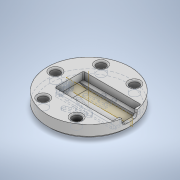
# Autodesk Inventor part: hmmb
Saved by Autodesk Inventor 2021 (Build 250183000, 183)
## iProperties
Created: 2020-07-09
Part Number: hmmb
Material: Generic
Document SubType Name: Modeling
Designer: andre
Density: 1 g/cm^3
Appearance: Default
Author: andre
## iProperties of the stored document _3DPrint.ipt
Created: 2020-07-09
Part Number: _3DPrint
Material: Generic
Document SubType Name: Modeling
Designer: andre
Density: 1 g/cm^3
Appearance: Default
Author: andre
Autodesk Inventor part; units mm, degrees
ref_plane "YZ Plane" through (0, 0, 0) normal (1, 0, 0) x (0, 1, 0)
ref_plane "XZ Plane" through (0, 0, 0) normal (0, 1, 0) x (-1, 0, 0)
ref_plane "XY Plane" through (0, 0, 0) normal (0, 0, 1) x (1, 0, 0)
sketch "Sketch1" plane through (0, 0, 0) normal (0, 1, 0) x (-1, 0, 0)
  circle A0 centre (0, 0) radius 26
  dimension "d0" = 52
  constraints: 1 centre point
  measures "d0" diameter of A0
extrude "Extrusion1" add sketch "Sketch1" along normal blind 8
chamfer "Chamfer2" distance 1.6 angle 45 1 edges at (26, 0, 0)
sketch "Sketch2" plane through (0, 8, 0) normal (0, 1, 0) x (1, 0, 0)
  line L0 (-12.4, -8.99) -> (23.96, -8.99)
  line L1 (23.96, -8.99) -> (23.96, 8.99)
  line L2 (23.96, 8.99) -> (-12.4, 8.99)
  line L3 (-12.4, 8.99) -> (-12.4, -8.99)
  point P0 (0, 0)
  dimension "d5" = 36.36
  dimension "d6" = 17.98
  dimension "d7" = 8.99
  dimension "d8" = 12.4
  constraints: 8 end point, 2 parallel, 1 horizontal, 1 perpendicular
  measures "d5" distance of L2.end L1.end
  measures "d6" distance of L1.end L0.end
  measures "d7" distance from line of point (0, 0) L2
  measures "d8" distance from line of point (0, 0) L3
extrude "Extrusion2" cut sketch "Sketch2" against normal blind 4.6
sketch "Sketch3" plane through (23.96, 8, -8.99) normal (-1, 0, 0) x (0, 0, 1)
  line L0 (4.2, 0) -> (13.78, 0)
  line L1 (13.78, 0) -> (13.78, -3.8)
  line L2 (13.78, -3.8) -> (4.2, -3.8)
  line L3 (4.2, -3.8) -> (4.2, 0)
  line L4 (0, 0) -> (17.98, 0) projected
  line L5 (0, -4.6) -> (17.98, -4.6) projected
  line L6 (0, 0) -> (0, -4.6) projected
  line L7 (17.98, 0) -> (17.98, -4.6) projected
  point P0 (8.99, -8)
  dimension "d11" = 0
  dimension "d14" = 4.2
  dimension "d44" = 4.2
  dimension "d47" = 0.8
  constraints: 8 end point, 2 parallel, 1 horizontal, 1 perpendicular
  measures "d11" distance between parallel lines of L4 L0
  measures "d14" distance between parallel lines of L7 L1
  measures "d44" distance between parallel lines of L6 L3
  measures "d47" distance between parallel lines of L5 L2
extrude "Extrusion3" cut sketch "Sketch3" against normal through all contours L0 L1 L2 L3
ref_plane "Work Plane1" through (-12.4, 8, 0) normal (0, 0, 1) x (1, 0, 0)
sketch "Sketch7" plane through (0, 3.4, 0) normal (0, 1, 0) x (1, 0, 0)
  line L0 (-12.4, 6.35) -> (23.16, 6.35)
  line L1 (23.16, 6.35) -> (23.16, -6.35)
  line L2 (23.16, -6.35) -> (-12.4, -6.35)
  line L3 (-12.4, -6.35) -> (-12.4, 6.35)
  line L4 (36.4, 0) -> (-36.4, 0) projected
  line L5 (-12.4, -8.99) -> (-12.4, 8.99) projected
  line L6 (23.96, -8.99) -> (-12.4, -8.99) projected
  point P0 (0, 0)
  dimension "d28" = 12.7
  dimension "d29" = 35.56
  dimension "d30" = 6.35
  dimension "d31" = 0
  dimension "d79" = 2.64
  constraints: 8 end point, 2 parallel, 1 horizontal, 1 perpendicular
  measures "d28" distance of L0.end L1.end
  measures "d29" distance between parallel lines of L1 L3
  measures "d30" distance between parallel lines of L4 L0
  measures "d31" distance between parallel lines of L5 L3
  measures "d79" distance between parallel lines of L6 L2
extrude "Extrusion5" cut sketch "Sketch7" against normal blind 1.6
sketch "Sketch4" plane through (0, 8, 0) normal (0, 1, 0) x (1, 0, 0)
  circle A0 centre (-21, 0) radius 2.8
  arc A1 (25.555, 4.79) -> (25.555, -4.79) centre (0, 0) ccw projected
  point P0 (24.6995, 8.12)
  point P1 (24.6995, -8.12)
  dimension "d17" = 5.6
  dimension "d23" = 21
  constraints: 1 centre point
  measures "d17" diameter of A0
  measures "d23" distance of A0.centre A1.centre
extrude "Extrusion4" cut sketch "Sketch4" against normal blind 5.2
fillet "Fillet4" radius 1 1 edges at (-23.8, 8, 0)
pattern_circular "Circular Pattern2" count 5 over 240 about axis through (0, 8, 0) along (0, 1, 0) of "Extrusion4", "Fillet4" both ways yes
chamfer "Chamfer3" distance 1.5 distance2 5 1 edges at (-12.4, 1.8, 0) measured on face at (-12.4, 2.3, 0)
fillet "Fillet7" radius 0.8 4 edges at (23.96, 5.7, -8.99) (23.96, 5.7, 8.99) (-12.4, 5.7, 8.99) (-12.4, 5.7, -8.99) curvature continuous yes
sketch "Sketch12" plane through (0, 0, 0) normal (0, -1, 0) x (1, 0, 0)
  line L0 (12.3547, 12.0872) -> (12.3547, -12.0872) construction
  line L1 (12.3547, -12.0872) -> (-12.3547, -12.0872) construction
  line L2 (-12.3547, -12.0872) -> (-12.3547, 12.0872) construction
  line L3 (-12.3547, 12.0872) -> (12.3547, 12.0872) construction
  spline S0 degree 2 poles (-6.9887, 9.9266) (-7, 9.452) (-6.4915, 8.8644) (-5.9379, 8.7062) knots 0 0 0 1 2 2 2
  line L4 (-5.9379, 8.7062) -> (-3.3503, 7.8023)
  line L5 (-3.3503, 7.8023) -> (-3.3503, 2.6949)
  line L6 (-3.3503, 2.6949) -> (-5.9605, 1.8023)
  spline S1 degree 2 poles (-5.9605, 1.8023) (-6.5028, 1.6441) (-7, 1.0452) (-6.9887, 0.548) knots 0 0 0 1 2 2 2
  spline S2 degree 2 poles (-6.9887, 0.548) (-6.9887, 0.0057) (-6.3672, -0.661) (-5.8701, -0.6723) knots 0 0 0 1 2 2 2
  spline S3 degree 2 poles (-5.8701, -0.6723) (-5.7006, -0.6723) (-5.3503, -0.5932) (-5.113, -0.5141) knots 0 0 0 1 2 2 2
  line L7 (-5.113, -0.5141) -> (5.678, 3.4633)
  spline S4 degree 2 poles (5.678, 3.4633) (6.3672, 3.7232) (7, 4.5819) (6.9887, 5.2599) knots 0 0 0 1 2 2 2
  spline S5 degree 2 poles (6.9887, 5.2599) (7, 5.9153) (6.3446, 6.7853) (5.6667, 7.0226) knots 0 0 0 1 2 2 2
  line L8 (5.6667, 7.0226) -> (-5.113, 10.9887)
  spline S6 degree 2 poles (-5.113, 10.9887) (-5.339, 11.0791) (-5.7232, 11.1582) (-5.8701, 11.1582) knots 0 0 0 1 2 2 2
  spline S7 degree 2 poles (-5.8701, 11.1582) (-6.3898, 11.1469) (-6.9887, 10.4915) (-6.9887, 9.9266) knots 0 0 0 1 2 2 2
  line L9 (-1.4181, 7.226) -> (4.4237, 5.3051)
  line L10 (4.4237, 5.3051) -> (4.4237, 5.2373)
  line L11 (4.4237, 5.2373) -> (-1.4181, 3.2938)
  line L12 (-1.4181, 3.2938) -> (-1.4181, 7.226)
  spline S8 degree 2 poles (-6.9887, -3.6667) (-6.9887, -4.2429) (-6.3333, -4.8757) (-5.7232, -4.887) knots 0 0 0 1 2 2 2
  line L13 (-5.7232, -4.887) -> (-1.2486, -4.887)
  line L14 (-1.2486, -4.887) -> (-1.2486, -9.7006)
  spline S9 degree 2 poles (-1.2486, -9.7006) (-1.2486, -10.1864) (-0.7288, -10.7627) (-0.2542, -10.774) knots 0 0 0 1 2 2 2
  spline S10 degree 2 poles (-0.2542, -10.774) (0.209, -10.7627) (0.7288, -10.1864) (0.7401, -9.7006) knots 0 0 0 1 2 2 2
  line L15 (0.7401, -9.7006) -> (0.7401, -4.887)
  line L16 (0.7401, -4.887) -> (4.774, -4.887)
  line L17 (4.774, -4.887) -> (4.774, -10.1977)
  spline S11 degree 2 poles (4.774, -10.1977) (4.774, -10.6949) (5.3164, -11.3051) (5.8023, -11.3164) knots 0 0 0 1 2 2 2
  spline S12 degree 2 poles (5.8023, -11.3164) (6.2768, -11.3051) (6.8305, -10.7062) (6.8305, -10.1977) knots 0 0 0 1 2 2 2
  line L18 (6.8305, -10.1977) -> (6.8305, -3.6667)
  spline S13 degree 2 poles (6.8305, -3.6667) (6.8305, -3.0904) (6.1638, -2.4463) (5.565, -2.435) knots 0 0 0 1 2 2 2
  line L19 (5.565, -2.435) -> (-5.7232, -2.435)
  spline S14 degree 2 poles (-5.7232, -2.435) (-6.3333, -2.4463) (-6.9887, -3.0904) (-6.9887, -3.6667) knots 0 0 0 1 2 2 2
  point P0 (0, 0)
  dimension "d80" = 24.1744
  dimension "d81" = 12.0872
  dimension "d82" = 24.7094
  dimension "d83" = 12.3547
  constraints: 2 other
  measures "d80" distance between parallel lines of L1 L3
  measures "d81" distance from line of point (0, 0) L1
  measures "d82" distance between parallel lines of L2 L0
  measures "d83" distance from line of point (0, 0) L2
extrude "Extrusion9" cut sketch "Sketch12" against normal blind 1
sketch "Sketch13" plane through (0, 0, 0) normal (0, -1, 0) x (1, 0, 0)
  line L0 (-12.1742, 6.9467) -> (-12.1742, -6.9467) construction
  line L1 (-12.1742, -6.9467) -> (-18.2711, -6.9467) construction
  line L2 (-18.2711, -6.9467) -> (-18.2711, 6.9467) construction
  line L3 (-18.2711, 6.9467) -> (-12.1742, 6.9467) construction
  line L4 (-36.4, 0) -> (36.4, 0) projected
  spline S0 degree 2 poles (-17.2291, 3.0821) (-17.2259, 2.8986) (-17.0069, 2.6828) (-16.8201, 2.6795) knots 0 0 0 1 2 2 2
  line L5 (-16.8201, 2.6795) -> (-13.6735, 2.6795)
  spline S1 degree 2 poles (-13.6735, 2.6795) (-13.461, 2.6828) (-13.2194, 2.9243) (-13.2162, 3.1433) knots 0 0 0 1 2 2 2
  spline S2 degree 2 poles (-13.2162, 3.1433) (-13.2162, 3.2657) (-13.2774, 3.4879) (-13.3708, 3.6264) knots 0 0 0 1 2 2 2
  line L6 (-13.3708, 3.6264) -> (-13.9054, 4.3994)
  spline S3 degree 2 poles (-13.9054, 4.3994) (-13.973, 4.4928) (-14.118, 4.5765) (-14.2114, 4.5765) knots 0 0 0 1 2 2 2
  spline S4 degree 2 poles (-14.2114, 4.5765) (-14.3434, 4.5733) (-14.5012, 4.4155) (-14.5012, 4.2899) knots 0 0 0 1 2 2 2
  spline S5 degree 2 poles (-14.5012, 4.2899) (-14.5012, 4.2287) (-14.469, 4.1288) (-14.4304, 4.0741) knots 0 0 0 1 2 2 2
  line L7 (-14.4304, 4.0741) -> (-14.031, 3.504)
  line L8 (-14.031, 3.504) -> (-14.031, 3.4879)
  line L9 (-14.031, 3.4879) -> (-16.8201, 3.4879)
  spline S6 degree 2 poles (-16.8201, 3.4879) (-17.0069, 3.4847) (-17.2259, 3.2657) (-17.2291, 3.0821) knots 0 0 0 1 2 2 2
  line L10 (-17.1711, 1.4267) -> (-17.1711, -0.7279)
  spline S7 degree 2 poles (-17.1711, -0.7279) (-17.1679, -0.8889) (-16.994, -1.066) (-16.8458, -1.066) knots 0 0 0 1 2 2 2
  spline S8 degree 2 poles (-16.8458, -1.066) (-16.6977, -1.066) (-16.5238, -0.8889) (-16.5238, -0.7279) knots 0 0 0 1 2 2 2
  line L11 (-16.5238, -0.7279) -> (-16.5238, 0.7407)
  line L12 (-16.5238, 0.7407) -> (-16.5077, 0.7407)
  line L13 (-16.5077, 0.7407) -> (-15.6961, -0.1031)
  spline S9 degree 2 poles (-15.6961, -0.1031) (-15.3998, -0.4187) (-14.9586, -0.8019) (-14.556, -0.9726) (-14.3241, -0.9726) knots 0 0 0 1 2 3 3 3
  spline S10 degree 2 poles (-14.3241, -0.9726) (-13.9859, -0.9694) (-13.4771, -0.6248) (-13.1937, -0.0064) (-13.1904, 0.409) knots 0 0 0 1 2 3 3 3
  spline S11 degree 2 poles (-13.1904, 0.409) (-13.1937, 0.7794) (-13.4288, 1.3398) (-13.8056, 1.7005) (-14.0246, 1.7681) knots 0 0 0 1 2 3 3 3
  spline S12 degree 2 poles (-14.0246, 1.7681) (-14.0664, 1.781) (-14.1534, 1.7971) (-14.1985, 1.7971) knots 0 0 0 1 2 2 2
  spline S13 degree 2 poles (-14.1985, 1.7971) (-14.3531, 1.7971) (-14.5302, 1.6135) (-14.5302, 1.4493) knots 0 0 0 1 2 2 2
  spline S14 degree 2 poles (-14.5302, 1.4493) (-14.5334, 1.3205) (-14.4143, 1.153) (-14.2951, 1.0886) knots 0 0 0 1 2 2 2
  spline S15 degree 2 poles (-14.2951, 1.0886) (-14.06, 0.9823) (-13.8249, 0.6538) (-13.8249, 0.4187) knots 0 0 0 1 2 2 2
  spline S16 degree 2 poles (-13.8249, 0.4187) (-13.8281, 0.1514) (-14.1309, -0.1739) (-14.3756, -0.1771) knots 0 0 0 1 2 2 2
  spline S17 degree 2 poles (-14.3756, -0.1771) (-14.5109, -0.1804) (-14.7653, -0.0773) (-15.0777, 0.1868) (-15.3064, 0.4251) knots 0 0 0 1 2 3 3 3
  line L14 (-15.3064, 0.4251) -> (-16.4143, 1.5878)
  spline S18 degree 2 poles (-16.4143, 1.5878) (-16.527, 1.7101) (-16.7106, 1.8132) (-16.8233, 1.81) knots 0 0 0 1 2 2 2
  spline S19 degree 2 poles (-16.8233, 1.81) (-16.9779, 1.81) (-17.1679, 1.62) (-17.1711, 1.4267) knots 0 0 0 1 2 2 2
  spline S20 degree 2 poles (-17.2581, -2.9758) (-17.2548, -3.43) (-16.965, -4.1095) (-16.4368, -4.4895) (-16.0793, -4.4928) knots 0 0 0 1 2 3 3 3
  spline S21 degree 2 poles (-16.0793, -4.4928) (-15.6767, -4.4863) (-15.1937, -3.9775) (-15.1486, -3.5362) knots 0 0 0 1 2 2 2
  line L15 (-15.1486, -3.5362) -> (-15.1325, -3.5362)
  spline S22 degree 2 poles (-15.1325, -3.5362) (-15.0616, -3.8873) (-14.5946, -4.3414) (-14.221, -4.3478) knots 0 0 0 1 2 2 2
  spline S23 degree 2 poles (-14.221, -4.3478) (-13.9086, -4.3446) (-13.4449, -4.0032) (-13.1937, -3.3849) (-13.1904, -2.9694) knots 0 0 0 1 2 3 3 3
  spline S24 degree 2 poles (-13.1904, -2.9694) (-13.1969, -2.4509) (-13.5962, -1.7971) (-13.8893, -1.6651) knots 0 0 0 1 2 2 2
  spline S25 degree 2 poles (-13.8893, -1.6651) (-13.9569, -1.6361) (-14.0825, -1.6071) (-14.1502, -1.6071) knots 0 0 0 1 2 2 2
  spline S26 degree 2 poles (-14.1502, -1.6071) (-14.3015, -1.6071) (-14.4787, -1.7778) (-14.4819, -1.9485) knots 0 0 0 1 2 2 2
  spline S27 degree 2 poles (-14.4819, -1.9485) (-14.4819, -2.0837) (-14.366, -2.2512) (-14.2307, -2.3156) knots 0 0 0 1 2 2 2
  spline S28 degree 2 poles (-14.2307, -2.3156) (-14.0246, -2.409) (-13.8152, -2.7279) (-13.8152, -2.9726) knots 0 0 0 1 2 2 2
  spline S29 degree 2 poles (-13.8152, -2.9726) (-13.8185, -3.2689) (-14.0986, -3.5749) (-14.337, -3.5749) knots 0 0 0 1 2 2 2
  spline S30 degree 2 poles (-14.337, -3.5749) (-14.5785, -3.5717) (-14.8748, -3.2142) (-14.878, -2.905) knots 0 0 0 1 2 2 2
  line L16 (-14.878, -2.905) -> (-14.878, -2.744)
  spline S31 degree 2 poles (-14.878, -2.744) (-14.878, -2.5958) (-15.0358, -2.4348) (-15.1647, -2.4348) knots 0 0 0 1 2 2 2
  spline S32 degree 2 poles (-15.1647, -2.4348) (-15.2999, -2.4348) (-15.4545, -2.5958) (-15.4577, -2.744) knots 0 0 0 1 2 2 2
  line L17 (-15.4577, -2.744) -> (-15.4577, -2.9147)
  spline S33 degree 2 poles (-15.4577, -2.9147) (-15.4577, -3.2721) (-15.7605, -3.6618) (-16.0471, -3.6618) knots 0 0 0 1 2 2 2
  spline S34 degree 2 poles (-16.0471, -3.6618) (-16.2919, -3.6586) (-16.5978, -3.2915) (-16.6011, -2.9887) knots 0 0 0 1 2 2 2
  spline S35 degree 2 poles (-16.6011, -2.9887) (-16.6011, -2.6892) (-16.3724, -2.3349) (-16.1663, -2.2351) knots 0 0 0 1 2 2 2
  spline S36 degree 2 poles (-16.1663, -2.2351) (-16.0568, -2.1771) (-15.9537, -2.0097) (-15.9537, -1.8905) knots 0 0 0 1 2 2 2
  spline S37 degree 2 poles (-15.9537, -1.8905) (-15.9569, -1.7198) (-16.1373, -1.533) (-16.2951, -1.5298) knots 0 0 0 1 2 2 2
  spline S38 degree 2 poles (-16.2951, -1.5298) (-16.3563, -1.5298) (-16.4851, -1.562) (-16.5528, -1.5942) knots 0 0 0 1 2 2 2
  spline S39 degree 2 poles (-16.5528, -1.5942) (-16.746, -1.6844) (-17.0648, -2.0515) (-17.2548, -2.6023) (-17.2581, -2.9758) knots 0 0 0 1 2 3 3 3
  point P0 (0, 0)
  dimension "d86" = 13.8935
  dimension "d87" = 6.9467
  constraints: 2 other
  measures "d86" distance between parallel lines of L1 L3
  measures "d87" distance between parallel lines of L4 L1
extrude "Extrusion10" cut sketch "Sketch13" against normal blind 4 contours L10 S19 S18 L14 S17 L4 L13 L12 L11 | L4 L11 S8 S7 L10 | L4 S17 S16 S10 S9 L13 | S16 S15 S14 S13 S12 S11 S10 L4 | S6 L9 L8 L7 S5 S4 S3 L6 S2 S1 L5 S0 | S39 S38 S37 S36 S35 S34 S33 L17 S32 S31 L16 S30 S29 S28 S27 S26 S25 S24 S23 S22 L15 S21 S20
fillet "Fillet9" radius 2 2 edges at (24.7575, 4.2, -4.79) (24.7575, 4.2, 4.79) curvature continuous yes
equation "\"d7\" = 0.5 * d6"
equation "\"d44\" = d14"
equation "\"d30\" = 0.5 * d28"
equation "\"d81\" = 0.5 * d80"
equation "\"d83\" = 0.5 * d82"
equation "\"d24\" = 0.5 * d6"
body "Solid1"
